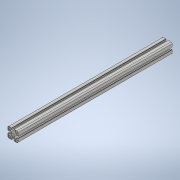
# Autodesk Inventor part: 2020 dai 300
Saved by Autodesk Inventor 2020 (Build 240168000, 168)
## iProperties
Created: 2020-04-28
Part Number: 2020 dai 300
Material: Generic
Document SubType Name: Modeling
Designer: Dell-T1700
Density: 1 g/cm^3
Appearance: Default
Author: Dell-T1700
Autodesk Inventor part; units mm, degrees
ref_plane "YZ Plane" through (0, 0, 0) normal (1, 0, 0) x (0, 1, 0)
ref_plane "XZ Plane" through (0, 0, 0) normal (0, 1, 0) x (-1, 0, 0)
ref_plane "XY Plane" through (0, 0, 0) normal (0, 0, 1) x (1, 0, 0)
sketch "Sketch1" plane through (0, 0, 0) normal (0, 0, 1) x (1, 0, 0)
  line L0 (-2.55, -10) -> (-2.55, -9.25)
  line L1 (-2.55, -9.25) -> (-2.05, -9.25)
  line L2 (-7.75, -10) -> (-2.55, -10)
  line L3 (-2.05, -9.25) -> (-2.05, -7)
  line L4 (-2.05, -7) -> (-3.05, -7)
  line L5 (-3.05, -9.1) -> (-3.05, -7)
  line L6 (-3.05, -9.1) -> (-5.125, -9.1)
  line L7 (-5.125, -9.1) -> (-5.125, -5.8321)
  line L8 (-8, -9.25) -> (-5.775, -9.25)
  line L9 (-5.775, -9.25) -> (-5.775, -5.775)
  line L10 (-2.2929, -3) -> (2.2929, -3)
  line L11 (3, -2.2929) -> (3, 2.2929)
  line L12 (2.2929, 3) -> (-2.2929, 3)
  line L13 (-3, 2.2929) -> (-3, -2.2929)
  line L14 (-2.2929, -3) -> (-5.125, -5.8321)
  line L15 (-3, -2.2929) -> (-5.8321, -5.125)
  line L16 (-9.1, -5.125) -> (-5.8321, -5.125)
  line L17 (-9.25, -5.775) -> (-5.775, -5.775)
  line L18 (-9.25, -8) -> (-9.25, -5.775)
  line L19 (-10, -7.75) -> (-10, -2.55)
  line L20 (-9.1, -3.05) -> (-9.1, -5.125)
  line L21 (-9.1, -3.05) -> (-7, -3.05)
  line L22 (-9.25, -2.55) -> (-9.25, -2.05)
  line L23 (-9.25, -2.05) -> (-7, -2.05)
  line L24 (-7, -2.05) -> (-7, -3.05)
  line L25 (-10, -2.55) -> (-9.25, -2.55)
  arc A0 (-9.25, -8) -> (-8, -9.25) centre (-8, -8) ccw
  arc A1 (-10, -7.75) -> (-7.75, -10) centre (-7.75, -7.75) ccw
  line L26 (3, -2.2929) -> (5.8321, -5.125)
  line L27 (2.2929, -3) -> (5.125, -5.8321)
  line L28 (5.775, -9.25) -> (5.775, -5.775)
  line L29 (8, -9.25) -> (5.775, -9.25)
  line L30 (7.75, -10) -> (2.55, -10)
  line L31 (3.05, -9.1) -> (5.125, -9.1)
  line L32 (2.55, -10) -> (2.55, -9.25)
  line L33 (3.05, -9.1) -> (3.05, -7)
  line L34 (2.05, -9.25) -> (2.05, -7)
  line L35 (2.55, -9.25) -> (2.05, -9.25)
  line L36 (2.05, -7) -> (3.05, -7)
  line L37 (5.125, -9.1) -> (5.125, -5.8321)
  arc A2 (8, -9.25) -> (9.25, -8) centre (8, -8) ccw
  arc A3 (7.75, -10) -> (10, -7.75) centre (7.75, -7.75) ccw
  line L38 (9.25, -8) -> (9.25, -5.775)
  line L39 (10, -7.75) -> (10, -2.55)
  line L40 (9.25, -5.775) -> (5.775, -5.775)
  line L41 (9.1, -5.125) -> (5.8321, -5.125)
  line L42 (9.1, -3.05) -> (7, -3.05)
  line L43 (7, -2.05) -> (7, -3.05)
  line L44 (9.25, -2.05) -> (7, -2.05)
  line L45 (9.25, -2.55) -> (9.25, -2.05)
  line L46 (10, -2.55) -> (9.25, -2.55)
  line L47 (9.1, -3.05) -> (9.1, -5.125)
  line L48 (2.2929, 3) -> (5.125, 5.8321)
  line L49 (3, 2.2929) -> (5.8321, 5.125)
  line L50 (9.25, 5.775) -> (5.775, 5.775)
  line L51 (9.25, 8) -> (9.25, 5.775)
  line L52 (10, 7.75) -> (10, 2.55)
  line L53 (9.1, 3.05) -> (9.1, 5.125)
  line L54 (10, 2.55) -> (9.25, 2.55)
  line L55 (9.1, 3.05) -> (7, 3.05)
  line L56 (9.25, 2.05) -> (7, 2.05)
  line L57 (9.25, 2.55) -> (9.25, 2.05)
  line L58 (7, 2.05) -> (7, 3.05)
  line L59 (9.1, 5.125) -> (5.8321, 5.125)
  arc A4 (9.25, 8) -> (8, 9.25) centre (8, 8) ccw
  arc A5 (10, 7.75) -> (7.75, 10) centre (7.75, 7.75) ccw
  line L60 (8, 9.25) -> (5.775, 9.25)
  line L61 (7.75, 10) -> (2.55, 10)
  line L62 (5.775, 9.25) -> (5.775, 5.775)
  line L63 (5.125, 9.1) -> (5.125, 5.8321)
  line L64 (3.05, 9.1) -> (3.05, 7)
  line L65 (2.05, 7) -> (3.05, 7)
  line L66 (2.05, 9.25) -> (2.05, 7)
  line L67 (2.55, 9.25) -> (2.05, 9.25)
  line L68 (2.55, 10) -> (2.55, 9.25)
  line L69 (3.05, 9.1) -> (5.125, 9.1)
  line L70 (-3, 2.2929) -> (-5.8321, 5.125)
  line L71 (-2.2929, 3) -> (-5.125, 5.8321)
  line L72 (-5.775, 9.25) -> (-5.775, 5.775)
  line L73 (-8, 9.25) -> (-5.775, 9.25)
  line L74 (-7.75, 10) -> (-2.55, 10)
  line L75 (-3.05, 9.1) -> (-5.125, 9.1)
  line L76 (-2.55, 10) -> (-2.55, 9.25)
  line L77 (-3.05, 9.1) -> (-3.05, 7)
  line L78 (-2.05, 9.25) -> (-2.05, 7)
  line L79 (-2.55, 9.25) -> (-2.05, 9.25)
  line L80 (-2.05, 7) -> (-3.05, 7)
  line L81 (-5.125, 9.1) -> (-5.125, 5.8321)
  arc A6 (-8, 9.25) -> (-9.25, 8) centre (-8, 8) ccw
  arc A7 (-7.75, 10) -> (-10, 7.75) centre (-7.75, 7.75) ccw
  line L82 (-9.25, 8) -> (-9.25, 5.775)
  line L83 (-10, 7.75) -> (-10, 2.55)
  line L84 (-9.25, 5.775) -> (-5.775, 5.775)
  line L85 (-9.1, 5.125) -> (-5.8321, 5.125)
  line L86 (-9.1, 3.05) -> (-7, 3.05)
  line L87 (-7, 2.05) -> (-7, 3.05)
  line L88 (-9.25, 2.05) -> (-7, 2.05)
  line L89 (-9.25, 2.55) -> (-9.25, 2.05)
  line L90 (-10, 2.55) -> (-9.25, 2.55)
  line L91 (-9.1, 3.05) -> (-9.1, 5.125)
  circle A8 centre (0, 0) radius 2
  point P0 (-10, -10)
  point P1 (10, -10)
  point P2 (10, 10)
  point P3 (-10, 10)
  dimension "d2" = 0.75
  dimension "d3" = 7.45
  dimension "d4" = 2.25
  dimension "d5" = 1
  dimension "d6" = 2.1
  dimension "d7" = 0.75
  dimension "d8" = 0.65
  dimension "d9" = 1.25
  dimension "d10" = 2.25
  dimension "d11" = 360
  dimension "d12" = 4
  dimension "d13" = 20
  constraints: 184 end point, 16 point on circle, 9 centre point, 8 point on line, 5 horizontal, 4 tangent, 3 perpendicular, 2 parallel, 2 vertical, 1 coincident, 209 other
  measures "d2" distance of L0.start L0.end
  measures "d3" distance of point (-10, -10) L0.start
  measures "d4" distance of L1.end L3.end
  measures "d5" distance of L3.end L4.end
  measures "d6" distance of L5.start L4.end
  measures "d7" distance between parallel lines of L2 L8
  measures "d8" distance between parallel lines of L7 L9
  measures "d9" radius of A0
  measures "d10" radius of A1
  measures "d12" diameter of A8
  measures "d13" distance between parallel lines of L83 L52
extrude "Extrusion1" add sketch "Sketch1" along normal blind 300
body "Solid1"
